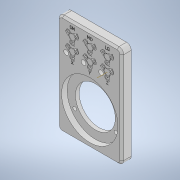
# Autodesk Inventor part: Case Front
Saved by Autodesk Inventor 2022 (Build 260153000, 153)
## iProperties
Created: 2022-10-09
Part Number: Case Front
Material: Generic
Document SubType Name: Modeling
Designer: Nick
Density: 1 g/cm^3
Appearance: Default
Author: Nick
Autodesk Inventor part; units mm, degrees
(part 1 of 2)
ref_plane "YZ Plane" through (0, 0, 0) normal (1, 0, 0) x (0, 1, 0)
ref_plane "XZ Plane" through (0, 0, 0) normal (0, 1, 0) x (-1, 0, 0)
ref_plane "XY Plane" through (0, 0, 0) normal (0, 0, 1) x (1, 0, 0)
sketch "Sketch1" plane through (0, 0, 0) normal (0, 0, 1) x (1, 0, 0)
  line L0 (0, 0) -> (68.58, 0)
  line L1 (68.58, 0) -> (68.58, 107.95)
  line L2 (68.58, 107.95) -> (0, 107.95)
  line L3 (0, 107.95) -> (0, 0)
  dimension "d0" = 68.58
  dimension "d1" = 107.95
  constraints: 8 end point, 2 parallel, 1 horizontal, 1 perpendicular
  measures "d0" distance of L2.end L1.end
  measures "d1" distance of L1.end L0.end
extrude "Extrusion1" add sketch "Sketch1" along normal blind 10
sketch "Sketch2" plane through (0, 0, 10) normal (0, 0, 1) x (1, 0, 0)
  circle A0 centre (34.29, 35.56) radius 30.099
  line L0 (0, 0) -> (68.58, 0) projected
  point P0 (34.29, 0)
  dimension "d4" = 60.198
  dimension "d5" = 35.56
  constraints: 1 centre point, 1 midpoint, 1 vertical alignment
  measures "d4" diameter of A0
  measures "d5" distance from line of L0 A0.centre
extrude "Extrusion2" cut sketch "Sketch2" against normal blind 16.9875
sketch "Sketch3" plane through (0, 0, 0) normal (0, 0, -1) x (-1, 0, 0)
  circle A0 centre (-34.29, 35.56) radius 30.099 projected
  circle A1 centre (-34.29, 35.56) radius 21.3106
  point P0 (0, 0)
  dimension "d8" = 42.6212
  constraints: 1 centre point, 1 coincident
  measures "d8" diameter of A1
extrude "Extrusion3" add sketch "Sketch3" against normal blind 4
sketch "Sketch4" plane through (0, 0, 10) normal (0, 0, 1) x (1, 0, 0)
  circle A0 centre (15.59, 79.9945) radius 3
  circle A1 centre (34.29, 79.9945) radius 3
  circle A2 centre (52.99, 93.6145) radius 3
  circle A3 centre (34.29, 93.6145) radius 3
  circle A4 centre (15.59, 93.6145) radius 3
  line L0 (12.59, 96.6145) -> (18.59, 96.6145) construction
  line L1 (18.59, 96.6145) -> (18.59, 90.6145) construction
  line L2 (18.59, 90.6145) -> (12.59, 90.6145) construction
  line L3 (12.59, 90.6145) -> (12.59, 96.6145) construction
  line L4 (31.29, 96.6145) -> (37.29, 96.6145) construction
  line L5 (37.29, 96.6145) -> (37.29, 90.6145) construction
  line L6 (37.29, 90.6145) -> (31.29, 90.6145) construction
  line L7 (31.29, 90.6145) -> (31.29, 96.6145) construction
  line L8 (49.99, 96.6145) -> (55.99, 96.6145) construction
  line L9 (55.99, 96.6145) -> (55.99, 90.6145) construction
  line L10 (55.99, 90.6145) -> (49.99, 90.6145) construction
  line L11 (49.99, 90.6145) -> (49.99, 96.6145) construction
  line L12 (31.29, 82.9945) -> (37.29, 82.9945) construction
  line L13 (37.29, 82.9945) -> (37.29, 76.9945) construction
  line L14 (37.29, 76.9945) -> (31.29, 76.9945) construction
  line L15 (31.29, 76.9945) -> (31.29, 82.9945) construction
  line L16 (12.59, 82.9945) -> (18.59, 82.9945) construction
  line L17 (18.59, 82.9945) -> (18.59, 76.9945) construction
  line L18 (18.59, 76.9945) -> (12.59, 76.9945) construction
  line L19 (12.59, 76.9945) -> (12.59, 82.9945) construction
  line L20 (68.58, 107.95) -> (0, 107.95) construction
  line L21 (17.8543, 65.659) -> (37.2658, 65.659) construction
  circle A5 centre (34.29, 35.56) radius 30.099 construction
  line L22 (27.9805, 81.0161) -> (29.433, 83.5319)
  line L23 (30.7639, 81.2971) -> (31.3989, 82.3969)
  line L24 (27.1145, 81.5161) -> (28.567, 84.0319)
  line L25 (29.8978, 81.7971) -> (30.5328, 82.8969)
  arc A6 (31.3989, 82.3969) -> (28.567, 84.0319) centre (29.9829, 83.2144) ccw
  arc A7 (30.5328, 82.8969) -> (29.433, 83.5319) centre (29.9829, 83.2144) ccw
  arc A8 (29.8978, 81.7971) -> (31.3611, 79.3453) centre (31.3138, 80.9796) ccw
  arc A9 (30.7639, 81.2971) -> (31.3105, 80.3446) centre (31.3138, 80.9796) ccw
  line L26 (34.29, 79.9945) -> (31.0814, 81.847) construction
  line L27 (34.29, 82.9945) -> (34.29, 79.9945) construction
  line L28 (27.1145, 81.5161) -> (27.9805, 81.0161)
  line L29 (26.6814, 81.7661) -> (28.4135, 80.7661)
  line L30 (28.4135, 80.7661) -> (29.866, 83.2819)
  line L31 (30.0998, 83.1469) -> (29.4648, 82.0471)
  arc A10 (30.0998, 83.1469) -> (29.866, 83.2819) centre (29.9829, 83.2144) ccw
  arc A11 (29.4648, 82.0471) -> (31.5152, 78.8541) centre (31.3138, 80.9796) ccw
  arc A12 (31.8319, 82.1469) -> (28.1339, 84.2819) centre (29.9829, 83.2144) ccw
  arc A13 (31.1969, 81.0471) -> (31.442, 80.9372) centre (31.3138, 80.9796) ccw
  line L32 (31.1969, 81.0471) -> (31.8319, 82.1469)
  line L33 (28.1339, 84.2819) -> (26.6814, 81.7661)
  circle A14 centre (52.99, 79.9945) radius 3
  line L34 (49.99, 82.9945) -> (55.99, 82.9945) construction
  line L35 (55.99, 82.9945) -> (55.99, 76.9945) construction
  line L36 (55.99, 76.9945) -> (49.99, 76.9945) construction
  line L37 (49.99, 76.9945) -> (49.99, 82.9945) construction
  line L38 (46.6805, 81.0161) -> (48.133, 83.5319)
  line L39 (49.4639, 81.2971) -> (50.0989, 82.3969)
  line L40 (45.8145, 81.5161) -> (47.267, 84.0319)
  line L41 (48.5978, 81.7971) -> (49.2328, 82.8969)
  arc A15 (50.0989, 82.3969) -> (47.267, 84.0319) centre (48.6829, 83.2144) ccw
  arc A16 (49.2328, 82.8969) -> (48.133, 83.5319) centre (48.6829, 83.2144) ccw
  arc A17 (48.5978, 81.7971) -> (50.0611, 79.3453) centre (50.0138, 80.9796) ccw
  arc A18 (49.4639, 81.2971) -> (50.0105, 80.3446) centre (50.0138, 80.9796) ccw
  line L42 (52.99, 79.9945) -> (49.7814, 81.847) construction
  line L43 (52.99, 82.9945) -> (52.99, 79.9945) construction
  line L44 (45.8145, 81.5161) -> (46.6805, 81.0161)
  line L45 (45.3814, 81.7661) -> (47.1135, 80.7661)
  line L46 (47.1135, 80.7661) -> (48.566, 83.2819)
  line L47 (48.7998, 83.1469) -> (48.1648, 82.0471)
  arc A19 (48.7998, 83.1469) -> (48.566, 83.2819) centre (48.6829, 83.2144) ccw
  arc A20 (48.1648, 82.0471) -> (50.2152, 78.8541) centre (50.0138, 80.9796) ccw
  arc A21 (50.5319, 82.1469) -> (46.8339, 84.2819) centre (48.6829, 83.2144) ccw
  arc A22 (49.8969, 81.0471) -> (50.142, 80.9372) centre (50.0138, 80.9796) ccw
  line L48 (49.8969, 81.0471) -> (50.5319, 82.1469)
  line L49 (46.8339, 84.2819) -> (45.3814, 81.7661)
  circle A23 centre (52.99, 79.9945) radius 3.508
  line L50 (47.1135, 80.7661) -> (48.557, 79.4188)
  point P0 (0, 0)
  point P1 (37.29, 79.9945)
  point P2 (18.59, 79.9945)
  point P3 (18.59, 93.6145)
  point P4 (31.29, 93.6145)
  point P5 (55.99, 93.6145)
  point P6 (34.29, 96.6145)
  point P7 (52.99, 96.6145)
  point P8 (15.59, 96.6145)
  point P9 (15.59, 82.9945)
  point P10 (34.29, 107.95)
  point P11 (27.5475, 81.2661)
  point P12 (55.99, 79.9945)
  point P13 (46.2475, 81.2661)
  point P14 (49.6661, 78.8731)
  point P15 (50.7545, 82.6979)
  point P16 (46.0107, 79.4247)
  dimension "d11" = 7.62
  dimension "d12" = 6
  dimension "d13" = 6
  dimension "d14" = 12.7
  dimension "d15" = 12.7
  dimension "d16" = 11.3355
  dimension "d17" = 11.3355
  dimension "d18" = 1
  dimension "d19" = 60
  dimension "d23" = 1.27
  dimension "d24" = 0.635
  dimension "d25" = 0.5
  dimension "d34" = 6
  dimension "d35" = 6
  dimension "d36" = 1
  dimension "d37" = 60
  dimension "d38" = 1.27
  dimension "d39" = 0.635
  dimension "d40" = 0.5
  dimension "d58" = 0.508
  constraints: 100 end point, 41 point on circle, 30 tangent, 26 parallel, 23 centre point, 19 midpoint, 12 concentric, 10 equal length, 10 perpendicular, 7 collinear, 7 horizontal, 7 vertical alignment, 6 equal radius, 6 horizontal alignment, 2 point on line, 2 vertical
  measures "d11" distance between parallel lines of L12 L6
  measures "d12" distance of L12.start L12.end
  measures "d13" diameter of A1
  measures "d14" distance between parallel lines of L11 L5
  measures "d15" distance between parallel lines of L1 L7
  measures "d16" distance between parallel lines of L20 L4
  measures "d17" distance between parallel lines of L21 L14
  measures "d18" distance between parallel lines of L23 L25
  measures "d19" angle of L27 L26
  measures "d23" distance of L25.start L25.end
  measures "d24" radius of A9
  measures "d25" distance between parallel lines of L30 L22
  measures "d34" distance of L37.end L35.start
  measures "d35" diameter of A14
  measures "d36" distance between parallel lines of L39 L41
  measures "d37" angle of L43 L42
  measures "d38" distance of L41.start L41.end
  measures "d39" radius of A18
  measures "d40" distance between parallel lines of L46 L38
  measures "d58" radial gap between concentric circles of A14 A23
extrude "Extrusion5" cut sketch "Sketch4" against normal through all contours A14 A18 A23 A21 L48 A22 | A20 A23 A17 A14 | A20 L47 A19 L46 L45 L38 A16 L41 A17 A23 | A18 L39 A15 L40 L45 L49 A21 A23 | L50 L46 A19 L47 A20
pattern_circular "Circular Pattern2" count 3 over 360 about axis through (52.99, 79.9945, 10) along (0, 0, 1) of "Extrusion5"
sketch "Sketch6" plane through (0, 0, 10) normal (0, 0, 1) x (1, 0, 0)
  arc A0 (53.8922, 82.8556) -> (53.3898, 82.9677) centre (52.99, 79.9945) ccw projected
  arc A1 (54.7079, 84.1214) -> (53.3898, 82.9677) centre (55.3312, 82.0794) ccw projected
  line L0 (56.5965, 84.6979) -> (57.0295, 84.9479) projected
  line L1 (57.0295, 84.9479) -> (58.482, 82.4321) projected
  arc A2 (57.3822, 81.7971) -> (58.482, 82.4321) centre (57.9321, 82.1146) ccw projected
  line L2 (57.3822, 81.7971) -> (56.7472, 82.8969) projected
  arc A3 (56.7472, 82.8969) -> (53.8922, 82.8556) centre (55.3312, 82.0794) ccw projected
  arc A4 (55.2304, 81.9897) -> (54.7829, 82.3998) centre (52.99, 79.9945) ccw projected
  arc A5 (55.8811, 82.3969) -> (54.7829, 82.3998) centre (55.3312, 82.0794) ccw projected
  line L3 (55.8811, 82.3969) -> (56.5161, 81.2971) projected
  arc A6 (56.5161, 81.2971) -> (59.348, 82.9321) centre (57.9321, 82.1146) ccw projected
  line L4 (59.348, 82.9321) -> (57.8955, 85.4479) projected
  line L5 (57.8955, 85.4479) -> (58.3286, 85.6979) projected
  line L6 (58.3286, 85.6979) -> (59.7811, 83.1821) projected
  arc A7 (56.0831, 81.0471) -> (59.7811, 83.1821) centre (57.9321, 82.1146) ccw projected
  line L7 (56.0831, 81.0471) -> (55.4481, 82.1469) projected
  arc A8 (55.4481, 82.1469) -> (55.2304, 81.9897) centre (55.3312, 82.0794) ccw projected
  arc A9 (55.0167, 77.7826) -> (55.365, 78.1617) centre (52.99, 79.9945) ccw projected
  arc A10 (55.7051, 76.4433) -> (55.365, 78.1617) centre (53.625, 76.9245) ccw projected
  line L8 (55.26, 74.5195) -> (55.26, 74.0195) projected
  line L9 (55.26, 74.0195) -> (52.355, 74.0195) projected
  arc A11 (52.355, 75.2895) -> (52.355, 74.0195) centre (52.355, 74.6545) ccw projected
  line L10 (52.355, 75.2895) -> (53.625, 75.2895) projected
  arc A12 (53.625, 75.2895) -> (55.0167, 77.7826) centre (53.625, 76.9245) ccw projected
  arc A13 (53.5977, 77.0567) -> (54.1766, 77.2391) centre (52.99, 79.9945) ccw projected
  arc A14 (53.625, 76.2895) -> (54.1766, 77.2391) centre (53.625, 76.9245) ccw projected
  line L11 (53.625, 76.2895) -> (52.355, 76.2895) projected
  arc A15 (52.355, 76.2895) -> (52.355, 73.0195) centre (52.355, 74.6545) ccw projected
  line L12 (52.355, 73.0195) -> (55.26, 73.0195) projected
  line L13 (55.26, 73.0195) -> (55.26, 72.5195) projected
  line L14 (55.26, 72.5195) -> (52.355, 72.5195) projected
  arc A16 (52.355, 76.7895) -> (52.355, 72.5195) centre (52.355, 74.6545) ccw projected
  line L15 (52.355, 76.7895) -> (53.625, 76.7895) projected
  arc A17 (53.625, 76.7895) -> (53.5977, 77.0567) centre (53.625, 76.9245) ccw projected
  line L16 (47.1135, 80.7661) -> (46.6805, 81.0161) projected
  line L17 (46.6805, 81.0161) -> (48.133, 83.5319) projected
  arc A18 (49.2328, 82.8969) -> (48.133, 83.5319) centre (48.6829, 83.2144) ccw projected
  line L18 (49.2328, 82.8969) -> (48.5978, 81.7971) projected
  arc A19 (48.5978, 81.7971) -> (50.0611, 79.3453) centre (50.0138, 80.9796) ccw projected
  arc A20 (50.0611, 79.3453) -> (50.2152, 78.8541) centre (52.99, 79.9945) ccw projected
  arc A21 (48.557, 79.4188) -> (50.2152, 78.8541) centre (50.0138, 80.9796) ccw projected
  line L19 (47.267, 84.0319) -> (45.8145, 81.5161) projected
  line L20 (45.8145, 81.5161) -> (45.3814, 81.7661) projected
  line L21 (45.3814, 81.7661) -> (46.8339, 84.2819) projected
  arc A22 (50.5319, 82.1469) -> (46.8339, 84.2819) centre (48.6829, 83.2144) ccw projected
  line L22 (50.5319, 82.1469) -> (49.8969, 81.0471) projected
  arc A23 (49.8969, 81.0471) -> (50.142, 80.9372) centre (50.0138, 80.9796) ccw projected
  arc A24 (50.142, 80.9372) -> (50.0105, 80.3446) centre (52.99, 79.9945) ccw projected
  arc A25 (49.4639, 81.2971) -> (50.0105, 80.3446) centre (50.0138, 80.9796) ccw projected
  line L23 (49.4639, 81.2971) -> (50.0989, 82.3969) projected
  arc A26 (50.0989, 82.3969) -> (47.267, 84.0319) centre (48.6829, 83.2144) ccw projected
  circle A27 centre (34.29, 35.56) radius 30.099 projected
  line L24 (68.58, 0) -> (68.58, 107.95) projected
  line L25 (68.58, 107.95) -> (0, 107.95) projected
  line L26 (0, 107.95) -> (0, 0) projected
  line L27 (0, 0) -> (68.58, 0) projected
  circle A28 centre (52.99, 79.9945) radius 3
  circle A29 centre (52.99, 79.9945) radius 3.508
  line L28 (54.7079, 84.1214) -> (56.5965, 84.6979) projected
  line L29 (55.7051, 76.4433) -> (55.26, 74.5195) projected
  line L30 (48.557, 79.4188) -> (47.1135, 80.7661) projected
  point P0 (53.5977, 77.0567)
  point P1 (50.2152, 78.8541)
  point P2 (49.6661, 78.8731)
  point P3 (51.7665, 76.7068)
  point P4 (55.2304, 81.9897)
  point P5 (55.365, 78.1617)
  point P6 (55.6231, 77.6766)
  point P7 (56.449, 80.5788)
  point P8 (50.142, 80.9372)
  point P9 (53.3898, 82.9677)
  point P10 (53.6808, 83.4338)
  point P11 (50.7545, 82.6979)
  dimension "d59" = 6
  dimension "d60" = 0.508
  constraints: 2 centre point, 1 coincident
  measures "d59" diameter of A28
  measures "d60" radial gap between concentric circles of A28 A29
extrude "Extrusion7" cut sketch "Sketch6" against normal through all contours A28 A23 L22 A22 A29 A1 | A8 L7 A7 A29 A10 A28 | A28 A17 L15 A16 A29 A21
pattern_linear "Rectangular Pattern2" count 3 spacing 18.7 along (-1, 0, 0) count 2 spacing 13.62 along (0, 1, 0) of "Extrusion5", "Circular Pattern2", "Extrusion7"
sketch "Sketch5" plane through (0, 0, 0) normal (0, 0, -1) x (-1, 0, 0)
  line L0 (-66.58, 105.95) -> (-2, 105.95)
  line L1 (-2, 105.95) -> (-2, 65.8874)
  line L2 (-2, 65.8874) -> (-66.58, 65.8874)
  line L3 (-66.58, 65.8874) -> (-66.58, 105.95)
  line L4 (-68.58, 107.95) -> (0, 107.95) projected
  line L5 (0, 107.95) -> (0, 0) projected
  line L6 (-68.58, 0) -> (-68.58, 107.95) projected
  line L7 (-14.955, 72.5195) -> (-17.86, 72.5195) projected
  point P0 (-20.9286, 99.3179)
  dimension "d52" = 2
  dimension "d53" = 2
  dimension "d54" = 2
  dimension "d74" = 6.6321
  dimension "d75" = 6.6321
  constraints: 8 end point, 2 parallel, 1 horizontal, 1 perpendicular
  measures "d52" distance between parallel lines of L4 L0
  measures "d53" distance between parallel lines of L5 L1
  measures "d54" distance between parallel lines of L6 L3
  measures "d74" distance from line of L0 point (-20.929, 99.318)
  measures "d75" distance between parallel lines of L2 L7
extrude "Extrusion6" cut sketch "Sketch5" against normal blind 9
sketch "Sketch7" plane through (0, 0, 10) normal (0, 0, 1) x (1, 0, 0)
  line L0 (11.8335, 71.5195) -> (19.3465, 71.5195) construction
  line L1 (19.3465, 71.5195) -> (19.3465, 68.4715) construction
  line L2 (19.3465, 68.4715) -> (11.8335, 68.4715) construction
  line L3 (11.8335, 68.4715) -> (11.8335, 71.5195) construction
  line L4 (30.5175, 71.5195) -> (38.0625, 71.5195) construction
  line L5 (38.0625, 71.5195) -> (38.0625, 68.4715) construction
  line L6 (38.0625, 68.4715) -> (30.5175, 68.4715) construction
  line L7 (30.5175, 68.4715) -> (30.5175, 71.5195) construction
  line L8 (54.358, 71.5195) -> (51.622, 71.5195) construction
  line L9 (51.622, 71.5195) -> (51.622, 68.4715) construction
  line L10 (51.622, 68.4715) -> (54.358, 68.4715) construction
  line L11 (54.358, 68.4715) -> (54.358, 71.5195) construction
  line L12 (12.8075, 103.4746) -> (18.3725, 103.4746) construction
  line L13 (18.3725, 103.4746) -> (18.3725, 100.3179) construction
  line L14 (18.3725, 100.3179) -> (12.8075, 100.3179) construction
  line L15 (12.8075, 100.3179) -> (12.8075, 103.4746) construction
  line L16 (31.2531, 103.3659) -> (37.3269, 103.3659) construction
  line L17 (37.3269, 103.3659) -> (37.3269, 100.3179) construction
  line L18 (37.3269, 100.3179) -> (31.2531, 100.3179) construction
  line L19 (31.2531, 100.3179) -> (31.2531, 103.3659) construction
  line L20 (50.5484, 103.4795) -> (55.4316, 103.4795) construction
  line L21 (55.4316, 103.4795) -> (55.4316, 100.3179) construction
  line L22 (55.4316, 100.3179) -> (50.5484, 100.3179) construction
  line L23 (50.5484, 100.3179) -> (50.5484, 103.4795) construction
  line L24 (68.58, 0) -> (68.58, 107.95) projected
  line L25 (68.58, 107.95) -> (0, 107.95) projected
  line L26 (0, 107.95) -> (0, 0) projected
  line L27 (0, 0) -> (68.58, 0) projected
  circle A0 centre (34.29, 35.56) radius 30.099 projected
  arc A1 (53.6808, 83.4338) -> (50.7545, 82.6979) centre (52.99, 79.9945) ccw projected
  arc A2 (54.7079, 84.1214) -> (53.6808, 83.4338) centre (55.3312, 82.0794) ccw projected
  line L28 (56.5965, 84.6979) -> (57.0295, 84.9479) projected
  line L29 (57.0295, 84.9479) -> (58.482, 82.4321) projected
  arc A3 (57.3822, 81.7971) -> (58.482, 82.4321) centre (57.9321, 82.1146) ccw projected
  line L30 (57.3822, 81.7971) -> (56.7472, 82.8969) projected
  arc A4 (56.7472, 82.8969) -> (53.8922, 82.8556) centre (55.3312, 82.0794) ccw projected
  arc A5 (53.8922, 82.8556) -> (50.0105, 80.3446) centre (52.99, 79.9945) ccw projected
  arc A6 (49.4639, 81.2971) -> (50.0105, 80.3446) centre (50.0138, 80.9796) ccw projected
  line L31 (49.4639, 81.2971) -> (50.0989, 82.3969) projected
  arc A7 (50.0989, 82.3969) -> (47.267, 84.0319) centre (48.6829, 83.2144) ccw projected
  line L32 (47.267, 84.0319) -> (45.8145, 81.5161) projected
  line L33 (45.8145, 81.5161) -> (45.3814, 81.7661) projected
  line L34 (45.3814, 81.7661) -> (46.8339, 84.2819) projected
  arc A8 (50.7545, 82.6979) -> (46.8339, 84.2819) centre (48.6829, 83.2144) ccw projected
  arc A9 (55.6231, 77.6766) -> (56.449, 80.5788) centre (52.99, 79.9945) ccw projected
  arc A10 (55.7051, 76.4433) -> (55.6231, 77.6766) centre (53.625, 76.9245) ccw projected
  line L35 (55.26, 74.5195) -> (55.26, 74.0195) projected
  line L36 (55.26, 74.0195) -> (52.355, 74.0195) projected
  arc A11 (52.355, 75.2895) -> (52.355, 74.0195) centre (52.355, 74.6545) ccw projected
  line L37 (52.355, 75.2895) -> (53.625, 75.2895) projected
  arc A12 (53.625, 75.2895) -> (55.0167, 77.7826) centre (53.625, 76.9245) ccw projected
  arc A13 (55.0167, 77.7826) -> (54.7829, 82.3998) centre (52.99, 79.9945) ccw projected
  arc A14 (55.8811, 82.3969) -> (54.7829, 82.3998) centre (55.3312, 82.0794) ccw projected
  line L38 (55.8811, 82.3969) -> (56.5161, 81.2971) projected
  arc A15 (56.5161, 81.2971) -> (59.348, 82.9321) centre (57.9321, 82.1146) ccw projected
  line L39 (59.348, 82.9321) -> (57.8955, 85.4479) projected
  line L40 (57.8955, 85.4479) -> (58.3286, 85.6979) projected
  line L41 (58.3286, 85.6979) -> (59.7811, 83.1821) projected
  arc A16 (56.449, 80.5788) -> (59.7811, 83.1821) centre (57.9321, 82.1146) ccw projected
  arc A17 (49.6661, 78.8731) -> (51.7665, 76.7068) centre (52.99, 79.9945) ccw projected
  arc A18 (48.557, 79.4188) -> (49.6661, 78.8731) centre (50.0138, 80.9796) ccw projected
  line L42 (47.1135, 80.7661) -> (46.6805, 81.0161) projected
  line L43 (46.6805, 81.0161) -> (48.133, 83.5319) projected
  arc A19 (49.2328, 82.8969) -> (48.133, 83.5319) centre (48.6829, 83.2144) ccw projected
  line L44 (49.2328, 82.8969) -> (48.5978, 81.7971) projected
  arc A20 (48.5978, 81.7971) -> (50.0611, 79.3453) centre (50.0138, 80.9796) ccw projected
  arc A21 (50.0611, 79.3453) -> (54.1766, 77.2391) centre (52.99, 79.9945) ccw projected
  arc A22 (53.625, 76.2895) -> (54.1766, 77.2391) centre (53.625, 76.9245) ccw projected
  line L45 (53.625, 76.2895) -> (52.355, 76.2895) projected
  arc A23 (52.355, 76.2895) -> (52.355, 73.0195) centre (52.355, 74.6545) ccw projected
  line L46 (52.355, 73.0195) -> (55.26, 73.0195) projected
  line L47 (55.26, 73.0195) -> (55.26, 72.5195) projected
  line L48 (55.26, 72.5195) -> (52.355, 72.5195) projected
  arc A24 (51.7665, 76.7068) -> (52.355, 72.5195) centre (52.355, 74.6545) ccw projected
  arc A25 (31.3611, 79.3453) -> (35.4766, 77.2391) centre (34.29, 79.9945) ccw projected
  arc A26 (34.925, 76.2895) -> (35.4766, 77.2391) centre (34.925, 76.9245) ccw projected
  line L49 (34.925, 76.2895) -> (33.655, 76.2895) projected
  arc A27 (33.655, 76.2895) -> (33.655, 73.0195) centre (33.655, 74.6545) ccw projected
  line L50 (33.655, 73.0195) -> (36.56, 73.0195) projected
  line L51 (36.56, 73.0195) -> (36.56, 72.5195) projected
  line L52 (36.56, 72.5195) -> (33.655, 72.5195) projected
  arc A28 (33.0665, 76.7068) -> (33.655, 72.5195) centre (33.655, 74.6545) ccw projected
  arc A29 (30.9661, 78.8731) -> (33.0665, 76.7068) centre (34.29, 79.9945) ccw projected
  arc A30 (29.857, 79.4188) -> (30.9661, 78.8731) centre (31.3138, 80.9796) ccw projected
  line L53 (28.4135, 80.7661) -> (27.9805, 81.0161) projected
  line L54 (27.9805, 81.0161) -> (29.433, 83.5319) projected
  arc A31 (30.5328, 82.8969) -> (29.433, 83.5319) centre (29.9829, 83.2144) ccw projected
  line L55 (30.5328, 82.8969) -> (29.8978, 81.7971) projected
  arc A32 (29.8978, 81.7971) -> (31.3611, 79.3453) centre (31.3138, 80.9796) ccw projected
  arc A33 (36.3167, 77.7826) -> (36.0829, 82.3998) centre (34.29, 79.9945) ccw projected
  arc A34 (37.1811, 82.3969) -> (36.0829, 82.3998) centre (36.6312, 82.0794) ccw projected
  line L56 (37.1811, 82.3969) -> (37.8161, 81.2971) projected
  arc A35 (37.8161, 81.2971) -> (40.648, 82.9321) centre (39.2321, 82.1146) ccw projected
  line L57 (40.648, 82.9321) -> (39.1955, 85.4479) projected
  line L58 (39.1955, 85.4479) -> (39.6286, 85.6979) projected
  line L59 (39.6286, 85.6979) -> (41.0811, 83.1821) projected
  arc A36 (37.749, 80.5788) -> (41.0811, 83.1821) centre (39.2321, 82.1146) ccw projected
  arc A37 (36.9231, 77.6766) -> (37.749, 80.5788) centre (34.29, 79.9945) ccw projected
  arc A38 (37.0051, 76.4433) -> (36.9231, 77.6766) centre (34.925, 76.9245) ccw projected
  line L60 (36.56, 74.5195) -> (36.56, 74.0195) projected
  line L61 (36.56, 74.0195) -> (33.655, 74.0195) projected
  arc A39 (33.655, 75.2895) -> (33.655, 74.0195) centre (33.655, 74.6545) ccw projected
  line L62 (33.655, 75.2895) -> (34.925, 75.2895) projected
  arc A40 (34.925, 75.2895) -> (36.3167, 77.7826) centre (34.925, 76.9245) ccw projected
  arc A41 (34.9808, 83.4338) -> (32.0545, 82.6979) centre (34.29, 79.9945) ccw projected
  arc A42 (36.0079, 84.1214) -> (34.9808, 83.4338) centre (36.6312, 82.0794) ccw projected
  line L63 (37.8965, 84.6979) -> (38.3295, 84.9479) projected
  line L64 (38.3295, 84.9479) -> (39.782, 82.4321) projected
  arc A43 (38.6822, 81.7971) -> (39.782, 82.4321) centre (39.2321, 82.1146) ccw projected
  line L65 (38.6822, 81.7971) -> (38.0472, 82.8969) projected
  arc A44 (38.0472, 82.8969) -> (35.1922, 82.8556) centre (36.6312, 82.0794) ccw projected
  arc A45 (35.1922, 82.8556) -> (31.3105, 80.3446) centre (34.29, 79.9945) ccw projected
  arc A46 (30.7639, 81.2971) -> (31.3105, 80.3446) centre (31.3138, 80.9796) ccw projected
  line L66 (30.7639, 81.2971) -> (31.3989, 82.3969) projected
  arc A47 (31.3989, 82.3969) -> (28.567, 84.0319) centre (29.9829, 83.2144) ccw projected
  line L67 (28.567, 84.0319) -> (27.1145, 81.5161) projected
  line L68 (27.1145, 81.5161) -> (26.6814, 81.7661) projected
  line L69 (26.6814, 81.7661) -> (28.1339, 84.2819) projected
  arc A48 (32.0545, 82.6979) -> (28.1339, 84.2819) centre (29.9829, 83.2144) ccw projected
  arc A49 (12.6611, 79.3453) -> (16.7766, 77.2391) centre (15.59, 79.9945) ccw projected
  arc A50 (16.225, 76.2895) -> (16.7766, 77.2391) centre (16.225, 76.9245) ccw projected
  line L70 (16.225, 76.2895) -> (14.955, 76.2895) projected
  arc A51 (14.955, 76.2895) -> (14.955, 73.0195) centre (14.955, 74.6545) ccw projected
  line L71 (14.955, 73.0195) -> (17.86, 73.0195) projected
  line L72 (17.86, 73.0195) -> (17.86, 72.5195) projected
  line L73 (17.86, 72.5195) -> (14.955, 72.5195) projected
  arc A52 (14.3665, 76.7068) -> (14.955, 72.5195) centre (14.955, 74.6545) ccw projected
  arc A53 (12.2661, 78.8731) -> (14.3665, 76.7068) centre (15.59, 79.9945) ccw projected
  arc A54 (11.157, 79.4188) -> (12.2661, 78.8731) centre (12.6138, 80.9796) ccw projected
  line L74 (9.7135, 80.7661) -> (9.2805, 81.0161) projected
  line L75 (9.2805, 81.0161) -> (10.733, 83.5319) projected
  arc A55 (11.8328, 82.8969) -> (10.733, 83.5319) centre (11.2829, 83.2144) ccw projected
  line L76 (11.8328, 82.8969) -> (11.1978, 81.7971) projected
  arc A56 (11.1978, 81.7971) -> (12.6611, 79.3453) centre (12.6138, 80.9796) ccw projected
  arc A57 (17.6167, 77.7826) -> (17.3829, 82.3998) centre (15.59, 79.9945) ccw projected
  arc A58 (18.4811, 82.3969) -> (17.3829, 82.3998) centre (17.9312, 82.0794) ccw projected
  line L77 (18.4811, 82.3969) -> (19.1161, 81.2971) projected
  arc A59 (19.1161, 81.2971) -> (21.948, 82.9321) centre (20.5321, 82.1146) ccw projected
  line L78 (21.948, 82.9321) -> (20.4955, 85.4479) projected
  line L79 (20.4955, 85.4479) -> (20.9286, 85.6979) projected
  line L80 (20.9286, 85.6979) -> (22.3811, 83.1821) projected
  arc A60 (19.049, 80.5788) -> (22.3811, 83.1821) centre (20.5321, 82.1146) ccw projected
  arc A61 (18.2231, 77.6766) -> (19.049, 80.5788) centre (15.59, 79.9945) ccw projected
  arc A62 (18.3051, 76.4433) -> (18.2231, 77.6766) centre (16.225, 76.9245) ccw projected
  line L81 (17.86, 74.5195) -> (17.86, 74.0195) projected
  line L82 (17.86, 74.0195) -> (14.955, 74.0195) projected
  arc A63 (14.955, 75.2895) -> (14.955, 74.0195) centre (14.955, 74.6545) ccw projected
  line L83 (14.955, 75.2895) -> (16.225, 75.2895) projected
  arc A64 (16.225, 75.2895) -> (17.6167, 77.7826) centre (16.225, 76.9245) ccw projected
  arc A65 (16.2808, 83.4338) -> (13.3545, 82.6979) centre (15.59, 79.9945) ccw projected
  arc A66 (17.3079, 84.1214) -> (16.2808, 83.4338) centre (17.9312, 82.0794) ccw projected
  line L84 (19.1965, 84.6979) -> (19.6295, 84.9479) projected
  line L85 (19.6295, 84.9479) -> (21.082, 82.4321) projected
  arc A67 (19.9822, 81.7971) -> (21.082, 82.4321) centre (20.5321, 82.1146) ccw projected
  line L86 (19.9822, 81.7971) -> (19.3472, 82.8969) projected
  arc A68 (19.3472, 82.8969) -> (16.4922, 82.8556) centre (17.9312, 82.0794) ccw projected
  arc A69 (16.4922, 82.8556) -> (12.6105, 80.3446) centre (15.59, 79.9945) ccw projected
  arc A70 (12.0639, 81.2971) -> (12.6105, 80.3446) centre (12.6138, 80.9796) ccw projected
  line L87 (12.0639, 81.2971) -> (12.6989, 82.3969) projected
  arc A71 (12.6989, 82.3969) -> (9.867, 84.0319) centre (11.2829, 83.2144) ccw projected
  line L88 (9.867, 84.0319) -> (8.4145, 81.5161) projected
  line L89 (8.4145, 81.5161) -> (7.9814, 81.7661) projected
  line L90 (7.9814, 81.7661) -> (9.4339, 84.2819) projected
  arc A72 (13.3545, 82.6979) -> (9.4339, 84.2819) centre (11.2829, 83.2144) ccw projected
  arc A73 (50.0611, 92.9653) -> (54.1766, 90.8591) centre (52.99, 93.6145) ccw projected
  arc A74 (53.625, 89.9095) -> (54.1766, 90.8591) centre (53.625, 90.5445) ccw projected
  line L91 (53.625, 89.9095) -> (52.355, 89.9095) projected
  arc A75 (52.355, 89.9095) -> (52.355, 86.6395) centre (52.355, 88.2745) ccw projected
  line L92 (52.355, 86.6395) -> (55.26, 86.6395) projected
  line L93 (55.26, 86.6395) -> (55.26, 86.1395) projected
  line L94 (55.26, 86.1395) -> (52.355, 86.1395) projected
  arc A76 (51.7665, 90.3268) -> (52.355, 86.1395) centre (52.355, 88.2745) ccw projected
  arc A77 (49.6661, 92.4931) -> (51.7665, 90.3268) centre (52.99, 93.6145) ccw projected
  arc A78 (48.557, 93.0388) -> (49.6661, 92.4931) centre (50.0138, 94.5996) ccw projected
  line L95 (47.1135, 94.3861) -> (46.6805, 94.6361) projected
  line L96 (46.6805, 94.6361) -> (48.133, 97.1519) projected
  arc A79 (49.2328, 96.5169) -> (48.133, 97.1519) centre (48.6829, 96.8344) ccw projected
  line L97 (49.2328, 96.5169) -> (48.5978, 95.4171) projected
  arc A80 (48.5978, 95.4171) -> (50.0611, 92.9653) centre (50.0138, 94.5996) ccw projected
  arc A81 (55.0167, 91.4026) -> (54.7829, 96.0198) centre (52.99, 93.6145) ccw projected
  arc A82 (55.8811, 96.0169) -> (54.7829, 96.0198) centre (55.3312, 95.6994) ccw projected
  line L98 (55.8811, 96.0169) -> (56.5161, 94.9171) projected
  arc A83 (56.5161, 94.9171) -> (59.348, 96.5521) centre (57.9321, 95.7346) ccw projected
  line L99 (59.348, 96.5521) -> (57.8955, 99.0679) projected
  line L100 (57.8955, 99.0679) -> (58.3286, 99.3179) projected
  line L101 (58.3286, 99.3179) -> (59.7811, 96.8021) projected
  arc A84 (56.449, 94.1988) -> (59.7811, 96.8021) centre (57.9321, 95.7346) ccw projected
  arc A85 (55.6231, 91.2966) -> (56.449, 94.1988) centre (52.99, 93.6145) ccw projected
  arc A86 (55.7051, 90.0633) -> (55.6231, 91.2966) centre (53.625, 90.5445) ccw projected
  line L102 (55.26, 88.1395) -> (55.26, 87.6395) projected
  line L103 (55.26, 87.6395) -> (52.355, 87.6395) projected
  arc A87 (52.355, 88.9095) -> (52.355, 87.6395) centre (52.355, 88.2745) ccw projected
  line L104 (52.355, 88.9095) -> (53.625, 88.9095) projected
  arc A88 (53.625, 88.9095) -> (55.0167, 91.4026) centre (53.625, 90.5445) ccw projected
  arc A89 (53.6808, 97.0538) -> (50.7545, 96.3179) centre (52.99, 93.6145) ccw projected
  arc A90 (54.7079, 97.7414) -> (53.6808, 97.0538) centre (55.3312, 95.6994) ccw projected
  line L105 (56.5965, 98.3179) -> (57.0295, 98.5679) projected
  line L106 (57.0295, 98.5679) -> (58.482, 96.0521) projected
  arc A91 (57.3822, 95.4171) -> (58.482, 96.0521) centre (57.9321, 95.7346) ccw projected
  line L107 (57.3822, 95.4171) -> (56.7472, 96.5169) projected
  arc A92 (56.7472, 96.5169) -> (53.8922, 96.4756) centre (55.3312, 95.6994) ccw projected
  arc A93 (53.8922, 96.4756) -> (50.0105, 93.9646) centre (52.99, 93.6145) ccw projected
  arc A94 (49.4639, 94.9171) -> (50.0105, 93.9646) centre (50.0138, 94.5996) ccw projected
  line L108 (49.4639, 94.9171) -> (50.0989, 96.0169) projected
  arc A95 (50.0989, 96.0169) -> (47.267, 97.6519) centre (48.6829, 96.8344) ccw projected
  line L109 (47.267, 97.6519) -> (45.8145, 95.1361) projected
  line L110 (45.8145, 95.1361) -> (45.3814, 95.3861) projected
  line L111 (45.3814, 95.3861) -> (46.8339, 97.9019) projected
  arc A96 (50.7545, 96.3179) -> (46.8339, 97.9019) centre (48.6829, 96.8344) ccw projected
  arc A97 (31.3611, 92.9653) -> (35.4766, 90.8591) centre (34.29, 93.6145) ccw projected
  arc A98 (34.925, 89.9095) -> (35.4766, 90.8591) centre (34.925, 90.5445) ccw projected
  line L112 (34.925, 89.9095) -> (33.655, 89.9095) projected
  arc A99 (33.655, 89.9095) -> (33.655, 86.6395) centre (33.655, 88.2745) ccw projected
  line L113 (33.655, 86.6395) -> (36.56, 86.6395) projected
  line L114 (36.56, 86.6395) -> (36.56, 86.1395) projected
  line L115 (36.56, 86.1395) -> (33.655, 86.1395) projected
  arc A100 (33.0665, 90.3268) -> (33.655, 86.1395) centre (33.655, 88.2745) ccw projected
  arc A101 (30.9661, 92.4931) -> (33.0665, 90.3268) centre (34.29, 93.6145) ccw projected
  arc A102 (29.857, 93.0388) -> (30.9661, 92.4931) centre (31.3138, 94.5996) ccw projected
  line L116 (28.4135, 94.3861) -> (27.9805, 94.6361) projected
  line L117 (27.9805, 94.6361) -> (29.433, 97.1519) projected
  arc A103 (30.5328, 96.5169) -> (29.433, 97.1519) centre (29.9829, 96.8344) ccw projected
  line L118 (30.5328, 96.5169) -> (29.8978, 95.4171) projected
  arc A104 (29.8978, 95.4171) -> (31.3611, 92.9653) centre (31.3138, 94.5996) ccw projected
  arc A105 (36.3167, 91.4026) -> (36.0829, 96.0198) centre (34.29, 93.6145) ccw projected
  arc A106 (37.1811, 96.0169) -> (36.0829, 96.0198) centre (36.6312, 95.6994) ccw projected
  line L119 (37.1811, 96.0169) -> (37.8161, 94.9171) projected
  arc A107 (37.8161, 94.9171) -> (40.648, 96.5521) centre (39.2321, 95.7346) ccw projected
  line L120 (40.648, 96.5521) -> (39.1955, 99.0679) projected
  line L121 (39.1955, 99.0679) -> (39.6286, 99.3179) projected
  line L122 (39.6286, 99.3179) -> (41.0811, 96.8021) projected
  arc A108 (37.749, 94.1988) -> (41.0811, 96.8021) centre (39.2321, 95.7346) ccw projected
  arc A109 (36.9231, 91.2966) -> (37.749, 94.1988) centre (34.29, 93.6145) ccw projected
  arc A110 (37.0051, 90.0633) -> (36.9231, 91.2966) centre (34.925, 90.5445) ccw projected
  line L123 (36.56, 88.1395) -> (36.56, 87.6395) projected
  line L124 (36.56, 87.6395) -> (33.655, 87.6395) projected
  arc A111 (33.655, 88.9095) -> (33.655, 87.6395) centre (33.655, 88.2745) ccw projected
  line L125 (33.655, 88.9095) -> (34.925, 88.9095) projected
  arc A112 (34.925, 88.9095) -> (36.3167, 91.4026) centre (34.925, 90.5445) ccw projected
  arc A113 (34.9808, 97.0538) -> (32.0545, 96.3179) centre (34.29, 93.6145) ccw projected
  arc A114 (36.0079, 97.7414) -> (34.9808, 97.0538) centre (36.6312, 95.6994) ccw projected
  line L126 (37.8965, 98.3179) -> (38.3295, 98.5679) projected
  line L127 (38.3295, 98.5679) -> (39.782, 96.0521) projected
  arc A115 (38.6822, 95.4171) -> (39.782, 96.0521) centre (39.2321, 95.7346) ccw projected
  line L128 (38.6822, 95.4171) -> (38.0472, 96.5169) projected
  arc A116 (38.0472, 96.5169) -> (35.1922, 96.4756) centre (36.6312, 95.6994) ccw projected
  arc A117 (35.1922, 96.4756) -> (31.3105, 93.9646) centre (34.29, 93.6145) ccw projected
  arc A118 (30.7639, 94.9171) -> (31.3105, 93.9646) centre (31.3138, 94.5996) ccw projected
  line L129 (30.7639, 94.9171) -> (31.3989, 96.0169) projected
  arc A119 (31.3989, 96.0169) -> (28.567, 97.6519) centre (29.9829, 96.8344) ccw projected
  line L130 (28.567, 97.6519) -> (27.1145, 95.1361) projected
  line L131 (27.1145, 95.1361) -> (26.6814, 95.3861) projected
  line L132 (26.6814, 95.3861) -> (28.1339, 97.9019) projected
  arc A120 (32.0545, 96.3179) -> (28.1339, 97.9019) centre (29.9829, 96.8344) ccw projected
  arc A121 (12.6611, 92.9653) -> (16.7766, 90.8591) centre (15.59, 93.6145) ccw projected
  arc A122 (16.225, 89.9095) -> (16.7766, 90.8591) centre (16.225, 90.5445) ccw projected
  line L133 (16.225, 89.9095) -> (14.955, 89.9095) projected
  arc A123 (14.955, 89.9095) -> (14.955, 86.6395) centre (14.955, 88.2745) ccw projected
  line L134 (14.955, 86.6395) -> (17.86, 86.6395) projected
  line L135 (17.86, 86.6395) -> (17.86, 86.1395) projected
  line L136 (17.86, 86.1395) -> (14.955, 86.1395) projected
  arc A124 (14.3665, 90.3268) -> (14.955, 86.1395) centre (14.955, 88.2745) ccw projected
  arc A125 (12.2661, 92.4931) -> (14.3665, 90.3268) centre (15.59, 93.6145) ccw projected
  arc A126 (11.157, 93.0388) -> (12.2661, 92.4931) centre (12.6138, 94.5996) ccw projected
  line L137 (9.7135, 94.3861) -> (9.2805, 94.6361) projected
  line L138 (9.2805, 94.6361) -> (10.733, 97.1519) projected
  arc A127 (11.8328, 96.5169) -> (10.733, 97.1519) centre (11.2829, 96.8344) ccw projected
  line L139 (11.8328, 96.5169) -> (11.1978, 95.4171) projected
  arc A128 (11.1978, 95.4171) -> (12.6611, 92.9653) centre (12.6138, 94.5996) ccw projected
  arc A129 (17.6167, 91.4026) -> (17.3829, 96.0198) centre (15.59, 93.6145) ccw projected
  arc A130 (18.4811, 96.0169) -> (17.3829, 96.0198) centre (17.9312, 95.6994) ccw projected
  line L140 (18.4811, 96.0169) -> (19.1161, 94.9171) projected
  arc A131 (19.1161, 94.9171) -> (21.948, 96.5521) centre (20.5321, 95.7346) ccw projected
  line L141 (21.948, 96.5521) -> (20.4955, 99.0679) projected
  line L142 (20.4955, 99.0679) -> (20.9286, 99.3179) projected
  line L143 (20.9286, 99.3179) -> (22.3811, 96.8021) projected
  arc A132 (19.049, 94.1988) -> (22.3811, 96.8021) centre (20.5321, 95.7346) ccw projected
  arc A133 (18.2231, 91.2966) -> (19.049, 94.1988) centre (15.59, 93.6145) ccw projected
  arc A134 (18.3051, 90.0633) -> (18.2231, 91.2966) centre (16.225, 90.5445) ccw projected
  line L144 (17.86, 88.1395) -> (17.86, 87.6395) projected
  line L145 (17.86, 87.6395) -> (14.955, 87.6395) projected
  arc A135 (14.955, 88.9095) -> (14.955, 87.6395) centre (14.955, 88.2745) ccw projected
  line L146 (14.955, 88.9095) -> (16.225, 88.9095) projected
  arc A136 (16.225, 88.9095) -> (17.6167, 91.4026) centre (16.225, 90.5445) ccw projected
  arc A137 (16.2808, 97.0538) -> (13.3545, 96.3179) centre (15.59, 93.6145) ccw projected
  arc A138 (17.3079, 97.7414) -> (16.2808, 97.0538) centre (17.9312, 95.6994) ccw projected
  line L147 (19.1965, 98.3179) -> (19.6295, 98.5679) projected
  line L148 (19.6295, 98.5679) -> (21.082, 96.0521) projected
  arc A139 (19.9822, 95.4171) -> (21.082, 96.0521) centre (20.5321, 95.7346) ccw projected
  line L149 (19.9822, 95.4171) -> (19.3472, 96.5169) projected
  arc A140 (19.3472, 96.5169) -> (16.4922, 96.4756) centre (17.9312, 95.6994) ccw projected
  arc A141 (16.4922, 96.4756) -> (12.6105, 93.9646) centre (15.59, 93.6145) ccw projected
  arc A142 (12.0639, 94.9171) -> (12.6105, 93.9646) centre (12.6138, 94.5996) ccw projected
  line L150 (12.0639, 94.9171) -> (12.6989, 96.0169) projected
  arc A143 (12.6989, 96.0169) -> (9.867, 97.6519) centre (11.2829, 96.8344) ccw projected
  line L151 (9.867, 97.6519) -> (8.4145, 95.1361) projected
  line L152 (8.4145, 95.1361) -> (7.9814, 95.3861) projected
  line L153 (7.9814, 95.3861) -> (9.4339, 97.9019) projected
  arc A144 (13.3545, 96.3179) -> (9.4339, 97.9019) centre (11.2829, 96.8344) ccw projected
  line L154 (54.7079, 84.1214) -> (56.5965, 84.6979) projected
  line L155 (55.7051, 76.4433) -> (55.26, 74.5195) projected
  line L156 (48.557, 79.4188) -> (47.1135, 80.7661) projected
  line L157 (29.857, 79.4188) -> (28.4135, 80.7661) projected
  line L158 (36.0079, 84.1214) -> (37.8965, 84.6979) projected
  line L159 (37.0051, 76.4433) -> (36.56, 74.5195) projected
  line L160 (11.157, 79.4188) -> (9.7135, 80.7661) projected
  line L161 (17.3079, 84.1214) -> (19.1965, 84.6979) projected
  line L162 (18.3051, 76.4433) -> (17.86, 74.5195) projected
  line L163 (48.557, 93.0388) -> (47.1135, 94.3861) projected
  line L164 (54.7079, 97.7414) -> (56.5965, 98.3179) projected
  line L165 (55.7051, 90.0633) -> (55.26, 88.1395) projected
  line L166 (29.857, 93.0388) -> (28.4135, 94.3861) projected
  line L167 (36.0079, 97.7414) -> (37.8965, 98.3179) projected
  line L168 (37.0051, 90.0633) -> (36.56, 88.1395) projected
  line L169 (11.157, 93.0388) -> (9.7135, 94.3861) projected
  line L170 (17.3079, 97.7414) -> (19.1965, 98.3179) projected
  line L171 (18.3051, 90.0633) -> (17.86, 88.1395) projected
  circle A145 centre (8.9909, 76.1845) radius 2.5
  circle A146 centre (27.6909, 76.1845) radius 2.5
  circle A147 centre (46.3909, 76.1845) radius 2.5
  line L172 (15.59, 79.9945) -> (52.99, 79.9945) construction
  arc A148 (31.3611, 79.3453) -> (35.4766, 77.2391) centre (34.29, 79.9945) ccw construction
  line L173 (34.29, 79.9945) -> (27.6909, 76.1845) construction
  line L174 (15.59, 79.9945) -> (8.9909, 76.1845) construction
  line L175 (52.99, 79.9945) -> (46.3909, 76.1845) construction
  spline S0 degree 2 poles (13.966, 100.3179) (13.635, 100.3179) (13.1706, 100.4562) (12.9656, 100.555) knots 0 0 0 1 2 2 2
  line L176 (12.9656, 100.555) -> (12.9656, 101.0638)
  line L177 (12.9656, 101.0638) -> (12.9952, 101.0638)
  spline S1 degree 2 poles (12.9952, 101.0638) (13.1953, 100.8761) (13.7017, 100.6686) (13.9363, 100.6686) knots 0 0 0 1 2 2 2
  spline S2 degree 2 poles (13.9363, 100.6686) (14.2722, 100.6686) (14.6156, 100.9477) (14.6156, 101.1775) knots 0 0 0 1 2 2 2
  spline S3 degree 2 poles (14.6156, 101.1775) (14.6156, 101.3602) (14.4353, 101.5875) (14.2401, 101.6443) knots 0 0 0 1 2 2 2
  spline S4 degree 2 poles (14.2401, 101.6443) (14.0993, 101.6838) (13.8647, 101.7381) (13.6893, 101.7826) knots 0 0 0 1 2 2 2
  spline S5 degree 2 poles (13.6893, 101.7826) (13.5312, 101.8246) (13.2818, 101.9506) (13.1854, 102.0518) knots 0 0 0 1 2 2 2
  spline S6 degree 2 poles (13.1854, 102.0518) (13.0916, 102.1531) (12.9878, 102.4248) (12.9878, 102.6027) knots 0 0 0 1 2 2 2
  spline S7 degree 2 poles (12.9878, 102.6027) (12.9878, 102.9732) (13.5658, 103.4746) (14.0129, 103.4746) knots 0 0 0 1 2 2 2
  spline S8 degree 2 poles (14.0129, 103.4746) (14.2698, 103.4746) (14.7243, 103.3733) (14.9194, 103.277) knots 0 0 0 1 2 2 2
  line L178 (14.9194, 103.277) -> (14.9194, 102.7928)
  line L179 (14.9194, 102.7928) -> (14.8898, 102.7928)
  spline S9 degree 2 poles (14.8898, 102.7928) (14.744, 102.9262) (14.2895, 103.1238) (14.0401, 103.1238) knots 0 0 0 1 2 2 2
  spline S10 degree 2 poles (14.0401, 103.1238) (13.7585, 103.1238) (13.4102, 102.8595) (13.4102, 102.6446) knots 0 0 0 1 2 2 2
  spline S11 degree 2 poles (13.4102, 102.6446) (13.4102, 102.452) (13.6152, 102.2223) (13.8079, 102.1704) knots 0 0 0 1 2 2 2
  spline S12 degree 2 poles (13.8079, 102.1704) (13.9363, 102.1358) (14.3093, 102.0469) (14.4328, 102.0098) knots 0 0 0 1 2 2 2
  spline S13 degree 2 poles (14.4328, 102.0098) (14.7465, 101.9135) (15.038, 101.5257) (15.038, 101.2417) knots 0 0 0 1 2 2 2
  spline S14 degree 2 poles (15.038, 101.2417) (15.038, 101.0614) (14.8922, 100.7156) (14.7613, 100.5945) knots 0 0 0 1 2 2 2
  spline S15 degree 2 poles (14.7613, 100.5945) (14.6156, 100.4611) (14.2451, 100.3179) (13.966, 100.3179) knots 0 0 0 1 2 2 2
  line L180 (18.0637, 100.3722) -> (17.6586, 100.3722)
  line L181 (17.6586, 100.3722) -> (17.6586, 102.9979)
  line L182 (17.6586, 102.9979) -> (16.8633, 101.212)
  line L183 (16.8633, 101.212) -> (16.6163, 101.212)
  line L184 (16.6163, 101.212) -> (15.8284, 102.9979)
  line L185 (15.8284, 102.9979) -> (15.8284, 100.3722)
  line L186 (15.8284, 100.3722) -> (15.4504, 100.3722)
  line L187 (15.4504, 100.3722) -> (15.4504, 103.4202)
  line L188 (15.4504, 103.4202) -> (16.0037, 103.4202)
  line L189 (16.0037, 103.4202) -> (16.7645, 101.7233)
  line L190 (16.7645, 101.7233) -> (17.5006, 103.4202)
  line L191 (17.5006, 103.4202) -> (18.0637, 103.4202)
  line L192 (18.0637, 103.4202) -> (18.0637, 100.3722)
  line L193 (34.1751, 100.3179) -> (33.7701, 100.3179)
  line L194 (33.7701, 100.3179) -> (33.7701, 102.9435)
  line L195 (33.7701, 102.9435) -> (32.9747, 101.1577)
  line L196 (32.9747, 101.1577) -> (32.7277, 101.1577)
  line L197 (32.7277, 101.1577) -> (31.9398, 102.9435)
  line L198 (31.9398, 102.9435) -> (31.9398, 100.3179)
  line L199 (31.9398, 100.3179) -> (31.5619, 100.3179)
  line L200 (31.5619, 100.3179) -> (31.5619, 103.3659)
  line L201 (31.5619, 103.3659) -> (32.1152, 103.3659)
  line L202 (32.1152, 103.3659) -> (32.8759, 101.669)
  line L203 (32.8759, 101.669) -> (33.612, 103.3659)
  line L204 (33.612, 103.3659) -> (34.1751, 103.3659)
  line L205 (34.1751, 103.3659) -> (34.1751, 100.3179)
  spline S16 degree 2 poles (37.196, 101.8394) (37.196, 101.422) (36.8576, 100.7501) (36.5735, 100.5624) knots 0 0 0 1 2 2 2
  spline S17 degree 2 poles (36.5735, 100.5624) (36.3413, 100.4167) (35.8646, 100.3179) (35.4941, 100.3179) knots 0 0 0 1 2 2 2
  line L206 (35.4941, 100.3179) -> (34.7926, 100.3179)
  line L207 (34.7926, 100.3179) -> (34.7926, 103.3659)
  line L208 (34.7926, 103.3659) -> (35.4867, 103.3659)
  spline S18 degree 2 poles (35.4867, 103.3659) (35.9165, 103.3659) (36.4056, 103.2374) (36.5785, 103.1238) knots 0 0 0 1 2 2 2
  spline S19 degree 2 poles (36.5785, 103.1238) (36.8724, 102.9287) (37.196, 102.284) (37.196, 101.8394) knots 0 0 0 1 2 2 2
  spline S20 degree 2 poles (36.7736, 101.8444) (36.7736, 102.1951) (36.5414, 102.6916) (36.3117, 102.8324) knots 0 0 0 1 2 2 2
  spline S21 degree 2 poles (36.3117, 102.8324) (36.1487, 102.9287) (35.7807, 103.0151) (35.5065, 103.0151) knots 0 0 0 1 2 2 2
  line L209 (35.5065, 103.0151) -> (35.1977, 103.0151)
  line L210 (35.1977, 103.0151) -> (35.1977, 100.6686)
  line L211 (35.1977, 100.6686) -> (35.5065, 100.6686)
  spline S22 degree 2 poles (35.5065, 100.6686) (35.7757, 100.6686) (36.1833, 100.7551) (36.3488, 100.8712) knots 0 0 0 1 2 2 2
  spline S23 degree 2 poles (36.3488, 100.8712) (36.5612, 101.0144) (36.7736, 101.4887) (36.7736, 101.8444) knots 0 0 0 1 2 2 2
  line L212 (52.6232, 100.3772) -> (50.8571, 100.3772)
  line L213 (50.8571, 100.3772) -> (50.8571, 103.4252)
  line L214 (50.8571, 103.4252) -> (51.2622, 103.4252)
  line L215 (51.2622, 103.4252) -> (51.2622, 100.7378)
  line L216 (51.2622, 100.7378) -> (52.6232, 100.7378)
  line L217 (52.6232, 100.7378) -> (52.6232, 100.3772)
  spline S24 degree 2 poles (54.2188, 100.3179) (53.8953, 100.3179) (53.3593, 100.5155) (53.1666, 100.7156) knots 0 0 0 1 2 2 2
  spline S25 degree 2 poles (53.1666, 100.7156) (52.9739, 100.9181) (52.7689, 101.5158) (52.7689, 101.9036) knots 0 0 0 1 2 2 2
  spline S26 degree 2 poles (52.7689, 101.9036) (52.7689, 102.2717) (52.9764, 102.8546) (53.1691, 103.0621) knots 0 0 0 1 2 2 2
  spline S27 degree 2 poles (53.1691, 103.0621) (53.3543, 103.2621) (53.8977, 103.4795) (54.2213, 103.4795) knots 0 0 0 1 2 2 2
  spline S28 degree 2 poles (54.2213, 103.4795) (54.3769, 103.4795) (54.6585, 103.435) (54.7869, 103.3955) knots 0 0 0 1 2 2 2
  spline S29 degree 2 poles (54.7869, 103.3955) (54.8907, 103.3659) (55.1426, 103.2572) (55.2192, 103.2177) knots 0 0 0 1 2 2 2
  line L218 (55.2192, 103.2177) -> (55.2192, 102.7286)
  line L219 (55.2192, 102.7286) -> (55.1846, 102.7286)
  spline S30 degree 2 poles (55.1846, 102.7286) (55.108, 102.7953) (54.9475, 102.9163) (54.7993, 102.9855) knots 0 0 0 1 2 2 2
  spline S31 degree 2 poles (54.7993, 102.9855) (54.6758, 103.0473) (54.3572, 103.1288) (54.1744, 103.1288) knots 0 0 0 1 2 2 2
  spline S32 degree 2 poles (54.1744, 103.1288) (53.7347, 103.1288) (53.1913, 102.4668) (53.1913, 101.916) knots 0 0 0 1 2 2 2
  spline S33 degree 2 poles (53.1913, 101.916) (53.1913, 101.6097) (53.3346, 101.1503) (53.4704, 100.9922) knots 0 0 0 1 2 2 2
  spline S34 degree 2 poles (53.4704, 100.9922) (53.6013, 100.8341) (53.9718, 100.6686) (54.204, 100.6686) knots 0 0 0 1 2 2 2
  spline S35 degree 2 poles (54.204, 100.6686) (54.3744, 100.6686) (54.7153, 100.718) (54.8314, 100.7674) knots 0 0 0 1 2 2 2
  line L220 (54.8314, 100.7674) -> (54.8314, 101.5554)
  line L221 (54.8314, 101.5554) -> (54.125, 101.5554)
  line L222 (54.125, 101.5554) -> (54.125, 101.911)
  line L223 (54.125, 101.911) -> (55.2315, 101.911)
  line L224 (55.2315, 101.911) -> (55.2315, 100.5797)
  spline S36 degree 2 poles (55.2315, 100.5797) (55.155, 100.5451) (54.8931, 100.4389) (54.782, 100.4068) knots 0 0 0 1 2 2 2
  spline S37 degree 2 poles (54.782, 100.4068) (54.6313, 100.3623) (54.3893, 100.3179) (54.2188, 100.3179) knots 0 0 0 1 2 2 2
  line L225 (16.7892, 68.4715) -> (16.3248, 68.4715)
  line L226 (16.3248, 68.4715) -> (15.5838, 69.6867)
  line L227 (15.5838, 69.6867) -> (14.828, 68.4715)
  line L228 (14.828, 68.4715) -> (14.3908, 68.4715)
  line L229 (14.3908, 68.4715) -> (15.3615, 69.998)
  line L230 (15.3615, 69.998) -> (14.4204, 71.5195)
  line L231 (14.4204, 71.5195) -> (14.8848, 71.5195)
  line L232 (14.8848, 71.5195) -> (15.611, 70.3265)
  line L233 (15.611, 70.3265) -> (16.352, 71.5195)
  line L234 (16.352, 71.5195) -> (16.7892, 71.5195)
  line L235 (16.7892, 71.5195) -> (15.8358, 70.0177)
  line L236 (15.8358, 70.0177) -> (16.7892, 68.4715)
  line L237 (35.5003, 71.5195) -> (34.4703, 69.8201)
  line L238 (34.4703, 69.8201) -> (34.4703, 68.4715)
  line L239 (34.4703, 68.4715) -> (34.0652, 68.4715)
  line L240 (34.0652, 68.4715) -> (34.0652, 69.7781)
  line L241 (34.0652, 69.7781) -> (33.0352, 71.5195)
  line L242 (33.0352, 71.5195) -> (33.4848, 71.5195)
  line L243 (33.4848, 71.5195) -> (34.2702, 70.1783)
  line L244 (34.2702, 70.1783) -> (35.0705, 71.5195)
  line L245 (35.0705, 71.5195) -> (35.5003, 71.5195)
  line L246 (51.9094, 71.5195) -> (54.0385, 71.5195)
  line L247 (54.0385, 71.5195) -> (54.0385, 71.1416)
  line L248 (54.0385, 71.1416) -> (52.4083, 68.8321)
  line L249 (52.4083, 68.8321) -> (53.9644, 68.8321)
  line L250 (53.9644, 68.8321) -> (53.9644, 68.4715)
  line L251 (53.9644, 68.4715) -> (51.9514, 68.4715)
  line L252 (51.9514, 68.4715) -> (51.9514, 68.837)
  line L253 (51.9514, 68.837) -> (53.5989, 71.1589)
  line L254 (53.5989, 71.1589) -> (51.9094, 71.1589)
  line L255 (51.9094, 71.1589) -> (51.9094, 71.5195)
  point P0 (52.99, 100.3179)
  point P1 (34.29, 100.3179)
  point P2 (15.59, 100.3179)
  point P3 (34.29, 79.9945)
  point P4 (34.29, 71.5195)
  point P5 (52.99, 71.5195)
  point P6 (15.59, 71.5195)
  dimension "d0" = 68.58
  dimension "d1" = 107.95
  dimension "d63" = 5
  dimension "d64" = 30
  dimension "d65" = 30
  dimension "d66" = 30
  dimension "d67" = 7.62
  dimension "d70" = 1
  dimension "d71" = 1
  constraints: 8 end point, 7 midpoint, 6 vertical alignment, 4 collinear, 3 centre point, 2 equal radius, 2 parallel, 1 horizontal, 12 other
  measures "d63" diameter of A145
  measures "d64" angle of L172 L175
  measures "d65" angle of L172 L173
  measures "d66" angle of L172 L174
  measures "d67" distance of L173.start L173.end
  measures "d70" distance between parallel lines of L52 L4
  measures "d71" distance from line of L121.end L18
extrude "Extrusion8" cut sketch "Sketch7" against normal through all contours A145 | A146 | A147
extrude "Extrusion9" cut sketch "Sketch7" against normal blind 0.5 contours S0 L176 L177 S1 S2 S3 S4 S5 S6 S7 S8 L178 L179 S9 S10 S11 S12 S13 S14 S15 | L180 L181 L182 L183 L184 L185 L186 L187 L188 L189 L190 L191 L192 | L193 L194 L195 L196 L197 L198 L199 L200 L201 L202 L203 L204 L205 | S16 S17 L206 L207 L208 S18 S19 | L212 L213 L214 L215 L216 L217 | S24 S25 S26 S27 S28 S29 L218 L219 S30 S31 S32 S33 S34 S35 L220 L221 L222 L223 L224 S36 S37 | L225 L226 L227 L228 L229 L230 L231 L232 L233 L234 L235 L236 | L237 L238 L239 L240 L241 L242 L243 L244 L245 | L246 L247 L248 L249 L250 L251 L252 L253 L254 L255